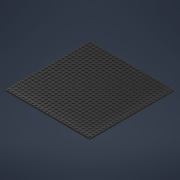
# Autodesk Inventor part: 110033226_ipt_36_瀑布基座
Saved by Autodesk Inventor 2022 (Build 260153000, 153)
## iProperties
Created: 2022-06-25
Part Number: 110033226_ipt_36_瀑布基座
Material: 一般
Document SubType Name: Modeling
Designer: User
Density: 1 g/cm^3
Appearance: 預設
Author: User
Autodesk Inventor part; units mm, degrees
ref_plane "YZ Plane" through (0, 0, 0) normal (1, 0, 0) x (0, 1, 0)
ref_plane "XZ Plane" through (0, 0, 0) normal (0, 1, 0) x (-1, 0, 0)
ref_plane "XY Plane" through (0, 0, 0) normal (0, 0, 1) x (1, 0, 0)
sketch "草圖1" plane through (0, 0, 0) normal (0, 1, 0) x (-1, 0, 0)
  line L0 (62.5, 62.5) -> (-62.5, 62.5)
  line L1 (-62.5, 62.5) -> (-62.5, -62.5)
  line L2 (-62.5, -62.5) -> (62.5, -62.5)
  line L3 (62.5, -62.5) -> (62.5, 62.5)
  point P0 (0, 0)
  point P1 (62.5, 0)
  point P2 (0, -62.5)
  dimension "d0" = 125
  dimension "d1" = 125
  constraints: 8 end point, 2 midpoint, 2 parallel, 1 horizontal, 1 horizontal alignment, 1 perpendicular, 1 vertical alignment
  measures "d0" distance of L2.end L1.end
  measures "d1" distance of L1.end L0.end
extrude "擠出1" add sketch "草圖1" along normal blind 2.5
sketch "草圖2" plane through (0, 2.5, 0) normal (0, 1, 0) x (1, 0, 0)
  circle A0 centre (-60, -60) radius 1.7
  line L0 (62.5, -62.5) -> (-62.5, -62.5) projected
  line L1 (-62.5, -62.5) -> (-62.5, 62.5) projected
  line L2 (-62.5, 62.5) -> (62.5, 62.5) projected
  line L3 (62.5, 62.5) -> (62.5, -62.5) projected
  point P0 (0, 0)
  dimension "d4" = 3.4
  dimension "d5" = 2.5
  dimension "d6" = 2.5
  constraints: 1 centre point
  measures "d4" diameter of A0
  measures "d5" distance from line of L1 A0.centre
  measures "d6" distance from line of L0 A0.centre
extrude "擠出2" add sketch "草圖2" along normal blind 1.5 contours A0
pattern_linear "矩形陣列1" count 25 spacing 5 along (0, 0, -1) count 25 spacing 5 along (1, 0, 0) of "擠出2"
sketch "草圖3" plane through (0, 0, 0) normal (0, -1, 0) x (1, 0, 0)
  line L0 (-62.5, 62.5) -> (62.5, 62.5) projected
  line L1 (62.5, 62.5) -> (62.5, -62.5) projected
  line L2 (62.5, -62.5) -> (-62.5, -62.5) projected
  line L3 (-62.5, -62.5) -> (-62.5, 62.5) projected
  circle A0 centre (-60, 60) radius 1.7 projected
  point P0 (0, 0)
extrude "擠出3" cut sketch "草圖3" against normal blind 1.5 contours A0
pattern_linear "矩形陣列2" count 25 spacing 5 along (1, 0, 0) count 25 spacing 5 along (0, 0, -1) of "擠出3"
